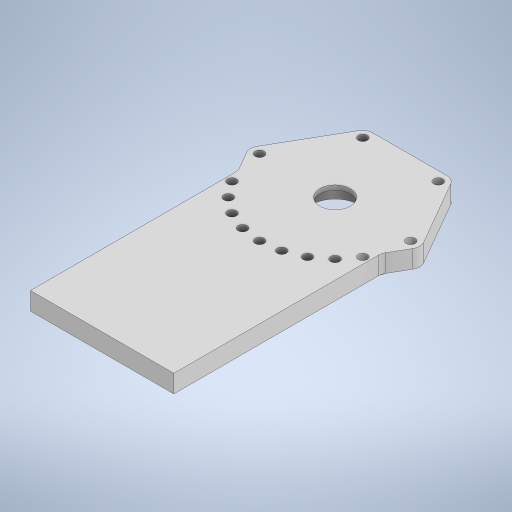
# Autodesk Inventor part: ZadKriska
Saved by Autodesk Inventor 2024 (Build 280153000, 153)
## iProperties
Created: 2023-08-25
Part Number: ZadKriska
Material: Generic
Document SubType Name: Modeling
Designer: KirikDK
Density: 1 g/cm^3
Appearance: Default
Author: KirikDK
Autodesk Inventor part; units mm, degrees
ref_plane "YZ Plane" through (0, 0, 0) normal (1, 0, 0) x (0, 1, 0)
ref_plane "XZ Plane" through (0, 0, 0) normal (0, 1, 0) x (-1, 0, 0)
ref_plane "XY Plane" through (0, 0, 0) normal (0, 0, 1) x (1, 0, 0)
sketch "Sketch1" plane through (0, 0, 0) normal (0, 1, 0) x (-1, 0, 0)
  line L0 (83.6786, 197.7945) -> (-76.3214, 197.7945)
  line L1 (-76.3214, 197.7945) -> (-76.3214, -52.2055)
  line L2 (-76.3214, -52.2055) -> (83.6786, -52.2055)
  line L3 (83.6786, -52.2055) -> (83.6786, 197.7945)
  circle A0 centre (3.6786, -62.2055) radius 80
  line L4 (83.6786, -52.2055) -> (83.6786, -62.2055)
  line L5 (-76.3214, -52.2055) -> (-76.3214, -62.2055)
  circle A1 centre (3.6786, -62.2055) radius 26
  circle A2 centre (3.6786, -62.2055) radius 40
  point P0 (0, 0)
  point P1 (59.3929, -23.6341)
  point P2 (-75.6939, -52.2055)
  point P3 (83.0512, -52.2055)
  dimension "d0" = 250
  dimension "d1" = 160
  dimension "d2" = 160
  dimension "d3" = 10
  dimension "d4" = 52
  dimension "d5" = 80
  constraints: 12 end point, 3 centre point, 2 coincident, 2 parallel, 2 point on circle, 1 horizontal, 1 perpendicular, 1 tangent, 1 vertical
  measures "d0" distance of L2.end L0.start
  measures "d1" distance of L0.start L0.end
  measures "d2" diameter of A0
  measures "d3" distance from line of A0.centre L2
  measures "d4" diameter of A1
  measures "d5" diameter of A2
extrude "Extrusion1" add sketch "Sketch1" along normal blind 20 contours L3 L2 A0 L1 L0 | L4 A0 L2 | L2 A0 L5 | A0 L2 A2 | L2 A2 A0 | A2 L2 A1 | L2 A1 A2
sketch "Sketch2" plane through (0, 20, 0) normal (0, 1, 0) x (1, 0, 0)
  circle A0 centre (-3.6786, 62.2055) radius 26 projected
  circle A1 centre (-3.6786, 62.2055) radius 26
  circle A2 centre (-3.6786, 62.2055) radius 17
  point P0 (0, 0)
  dimension "d8" = 34
  constraints: 2 centre point, 2 coincident
  measures "d8" diameter of A2
extrude "Extrusion2" add sketch "Sketch2" against normal blind 5
sketch "Sketch3" plane through (0, 0, 0) normal (0, -1, 0) x (1, 0, 0)
  circle A0 centre (-3.6786, -62.2055) radius 75
  circle A1 centre (-3.6786, -62.2055) radius 75
  line L0 (92.6071, -62.2055) -> (44.4642, -145.5914)
  line L1 (44.4642, -145.5914) -> (-51.8215, -145.5914)
  line L2 (-51.8215, -145.5914) -> (-99.9643, -62.2055)
  line L3 (-99.9643, -62.2055) -> (-51.8215, 21.1804)
  line L4 (-51.8215, 21.1804) -> (44.4642, 21.1804)
  line L5 (44.4642, 21.1804) -> (92.6071, -62.2055)
  line L6 (80.6071, -62.2055) -> (38.4642, -135.1991)
  line L7 (38.4642, -135.1991) -> (-45.8215, -135.1991)
  line L8 (-45.8215, -135.1991) -> (-87.9643, -62.2055)
  line L9 (-87.9643, -62.2055) -> (-45.8215, 10.7881)
  line L10 (-45.8215, 10.7881) -> (38.4642, 10.7881)
  line L11 (38.4642, 10.7881) -> (80.6071, -62.2055)
  circle A2 centre (80.6071, -62.2055) radius 5
  circle A3 centre (38.4642, 10.7881) radius 5
  circle A4 centre (-45.8215, 10.7881) radius 5
  circle A5 centre (-87.9643, -62.2055) radius 5
  circle A6 centre (-45.8215, -135.1991) radius 5
  circle A7 centre (38.4642, -135.1991) radius 5
  circle A8 centre (-3.6786, -62.2055) radius 26 projected
  circle A9 centre (-3.6786, -62.2055) radius 0.8535
  point P0 (0, 0)
  point P1 (-59.3929, -100.7769)
  point P2 (-3.6786, -62.2055)
  dimension "d13" = 360
  constraints: 24 end point, 9 centre point, 5 coincident, 39 other
sketch "Sketch4" plane through (0, 0, 0) normal (0, -1, 0) x (1, 0, 0)
  circle A0 centre (-45.8215, -135.1991) radius 5
  line L0 (-45.8215, -135.1991) -> (-87.9643, -62.2055)
  line L1 (-51.8215, -145.5914) -> (-99.9643, -62.2055)
  circle A1 centre (-87.9643, -62.2055) radius 5
  circle A2 centre (-45.8215, 10.7881) radius 5
  line L2 (-87.9643, -62.2055) -> (-45.8215, 10.7881)
  line L3 (-99.9643, -62.2055) -> (-51.8215, 21.1804)
  line L4 (38.4642, -135.1991) -> (-45.8215, -135.1991)
  circle A3 centre (38.4642, -135.1991) radius 5
  line L5 (44.4642, -145.5914) -> (-51.8215, -145.5914)
  line L6 (80.6071, -62.2055) -> (38.4642, -135.1991)
  line L7 (92.6071, -62.2055) -> (44.4642, -145.5914)
  circle A4 centre (-3.6786, -62.2055) radius 75
  circle A5 centre (-3.6786, -62.2055) radius 75
  line L8 (-45.8215, 10.7881) -> (38.4642, 10.7881)
  line L9 (-51.8215, 21.1804) -> (44.4642, 21.1804)
  circle A6 centre (80.6071, -62.2055) radius 5
  circle A7 centre (38.4642, 10.7881) radius 5
  line L10 (38.4642, 10.7881) -> (80.6071, -62.2055)
  line L11 (44.4642, 21.1804) -> (92.6071, -62.2055)
  circle A8 centre (-3.6786, -62.2055) radius 26
  circle A9 centre (-3.6786, -62.2055) radius 17 projected
  circle A10 centre (-3.6786, -62.2055) radius 2.3214
  point P0 (0, 0)
  point P1 (0, 0)
  point P2 (-59.3929, -100.7769)
  dimension "d18" = 360
  constraints: 24 end point, 10 centre point, 5 coincident, 39 other
extrude "Extrusion3" cut sketch "Sketch3" against normal blind 22 contours A2 L6 L11 | L11 L6 A2 | A3 L10 L11 | L11 L10 A3 | A7 L7 L6 | L6 L7 A7 | A4 L9 L10 | L10 L9 A4 | A6 L8 L7 | L7 L8 A6 | A5 L8 L9 | L9 L8 A5
extrude "Extrusion4" add sketch "Sketch4" against normal blind 20 contours A0 L0 A4 L4 | A4 L6 A3 L4 | L0 A1 L2 A4 | A4 L10 A6 L6 | L2 A2 L8 A4 | L8 A7 L10 A4 | L1 L3 L9 L11 L7 L5
sketch "Sketch5" plane through (0, 0, 0) normal (0, -1, 0) x (1, 0, 0)
  circle A0 centre (-3.6786, -62.2055) radius 17 projected
  circle A1 centre (-3.6786, -62.2055) radius 79.2857
  circle A2 centre (80.6071, -62.2055) radius 5 projected
  circle A3 centre (-3.6786, -62.2055) radius 75
  point P0 (0, 0)
  dimension "d21" = 150
  constraints: 2 centre point, 2 coincident, 1 tangent
  measures "d21" diameter of A3
extrude "Extrusion5" add sketch "Sketch5" along normal blind 5 contours A1
fillet "Fillet1" radius 12 6 edges at (-83.6786, 10, -33.9978) (-99.9643, 10, -62.2055) (-51.8215, 10, -145.5914) (44.4642, 10, -145.5914) (92.6071, 10, -62.2055) (76.3214, 10, -33.9978)
sketch "Sketch6" plane through (0, 0, 0) normal (0, -1, 0) x (1, 0, 0)
  arc A0 (89.143, -68.2055) -> (89.143, -56.2055) centre (78.7507, -62.2055) ccw projected
  line L0 (89.143, -56.2055) -> (77.9291, -36.7824) projected
  arc A1 (76.3214, -30.7824) -> (77.9291, -36.7824) centre (88.3214, -30.7824) ccw projected
  line L1 (76.3214, 197.7945) -> (76.3214, -30.7824) projected
  line L2 (-83.6786, 197.7945) -> (76.3214, 197.7945) projected
  line L3 (-83.6786, -30.7824) -> (-83.6786, 197.7945) projected
  arc A2 (-85.2863, -36.7824) -> (-83.6786, -30.7824) centre (-95.6786, -30.7824) ccw projected
  line L4 (-85.2863, -36.7824) -> (-96.5002, -56.2055) projected
  arc A3 (-96.5002, -56.2055) -> (-96.5002, -68.2055) centre (-86.1079, -62.2055) ccw projected
  line L5 (-96.5002, -68.2055) -> (-55.2856, -139.5914) projected
  arc A4 (-55.2856, -139.5914) -> (-44.8933, -145.5914) centre (-44.8933, -133.5914) ccw projected
  line L6 (-44.8933, -145.5914) -> (37.536, -145.5914) projected
  arc A5 (37.536, -145.5914) -> (47.9283, -139.5914) centre (37.536, -133.5914) ccw projected
  line L7 (47.9283, -139.5914) -> (89.143, -68.2055) projected
  circle A6 centre (-87.9643, -62.2055) radius 5 projected
  arc A7 (-43.3215, 6.4579) -> (-82.9643, -62.2055) centre (-3.6786, -62.2055) ccw projected
  circle A8 centre (-45.8215, 10.7881) radius 5 projected
  arc A9 (35.9642, 6.4579) -> (-43.3215, 6.4579) centre (-3.6786, -62.2055) ccw projected
  circle A10 centre (38.4642, 10.7881) radius 5 projected
  arc A11 (75.6071, -62.2055) -> (35.9642, 6.4579) centre (-3.6786, -62.2055) ccw projected
  circle A12 centre (80.6071, -62.2055) radius 5 projected
  arc A13 (35.9642, -130.869) -> (75.6071, -62.2055) centre (-3.6786, -62.2055) ccw projected
  circle A14 centre (38.4642, -135.1991) radius 5 projected
  arc A15 (-43.3215, -130.869) -> (35.9642, -130.869) centre (-3.6786, -62.2055) ccw projected
  circle A16 centre (-45.8215, -135.1991) radius 5 projected
  arc A17 (-82.9643, -62.2055) -> (-43.3215, -130.869) centre (-3.6786, -62.2055) ccw projected
  arc A18 (56.3214, -30.7824) -> (60.6086, -46.7824) centre (88.3214, -30.7824) ccw
  line L8 (60.6086, -46.7824) -> (69.5131, -62.2055)
  line L9 (69.5131, -62.2055) -> (32.9172, -125.5914)
  line L10 (32.9172, -125.5914) -> (-40.2745, -125.5914)
  line L11 (-40.2745, -125.5914) -> (-76.8703, -62.2055)
  line L12 (-76.8703, -62.2055) -> (-67.9658, -46.7824)
  arc A19 (-67.9658, -46.7824) -> (-63.6786, -30.7824) centre (-95.6786, -30.7824) ccw
  line L13 (-63.6786, -30.7824) -> (-63.6786, 177.7945)
  line L14 (-63.6786, 177.7945) -> (56.3214, 177.7945)
  line L15 (56.3214, 177.7945) -> (56.3214, -30.7824)
  arc A20 (-53.3215, 23.7784) -> (-102.9643, -62.2055) centre (-3.6786, -62.2055) ccw
  arc A21 (-102.9643, -62.2055) -> (-53.3215, -148.1895) centre (-3.6786, -62.2055) ccw
  arc A22 (-53.3215, -148.1895) -> (45.9642, -148.1895) centre (-3.6786, -62.2055) ccw
  arc A23 (45.9642, -148.1895) -> (95.6071, -62.2055) centre (-3.6786, -62.2055) ccw
  arc A24 (95.6071, -62.2055) -> (45.9642, 23.7784) centre (-3.6786, -62.2055) ccw
  arc A25 (45.9642, 23.7784) -> (-53.3215, 23.7784) centre (-3.6786, -62.2055) ccw
  point P0 (0, 0)
  point P1 (-63.6786, 16.8998)
  point P2 (56.3214, 16.8998)
  dimension "d25" = 20
  dimension "d26" = 20
  constraints: 16 end point, 16 point on circle, 8 centre point, 2 horizontal alignment, 18 other
  measures "d25" distance between parallel lines of L1 L15
  measures "d26" radial gap between concentric circles of A9 A25
extrude "Extrusion6" cut sketch "Sketch6" against normal blind 12 contours A24 A25 A20 L13 L14 L15
sketch "Sketch7" plane through (0, 0, 0) normal (0, -1, 0) x (1, 0, 0)
  circle A0 centre (-3.6786, 22.0805) radius 5
  circle A1 centre (-3.6786, -62.2055) radius 17 projected
  circle A2 centre (-25.4934, 19.2085) radius 5
  circle A3 centre (-45.8216, 10.7883) radius 5
  circle A4 centre (-63.2778, -2.6063) radius 5
  circle A5 centre (-76.6724, -20.0625) radius 5
  circle A6 centre (-85.0926, -40.3907) radius 5
  circle A7 centre (-87.9646, -62.2055) radius 5
  circle A8 centre (-85.0926, -84.0203) radius 5
  circle A9 centre (-76.6724, -104.3485) radius 5
  circle A10 centre (-63.2778, -121.8047) radius 5
  circle A11 centre (-45.8216, -135.1993) radius 5
  circle A12 centre (-25.4934, -143.6195) radius 5
  circle A13 centre (-3.6786, -146.4915) radius 5
  circle A14 centre (18.1362, -143.6195) radius 5
  circle A15 centre (38.4644, -135.1993) radius 5
  circle A16 centre (55.9206, -121.8047) radius 5
  circle A17 centre (69.3152, -104.3485) radius 5
  circle A18 centre (77.7354, -84.0203) radius 5
  circle A19 centre (80.6074, -62.2055) radius 5
  circle A20 centre (77.7354, -40.3907) radius 5
  circle A21 centre (69.3152, -20.0625) radius 5
  circle A22 centre (55.9206, -2.6063) radius 5
  circle A23 centre (38.4644, 10.7883) radius 5
  circle A24 centre (18.1362, 19.2085) radius 5
  point P0 (0, 0)
  dimension "d29" = 84.286
  dimension "d30" = 10
  dimension "d33" = 360
  constraints: 24 centre point, 49 other
  measures "d29" distance of A1.centre A0.centre
  measures "d30" diameter of A0
extrude "Extrusion7" cut sketch "Sketch7" against normal blind 39 contours A0 | A2 | A4 | A5 | A21 | A22 | A24
body "Solid1"
